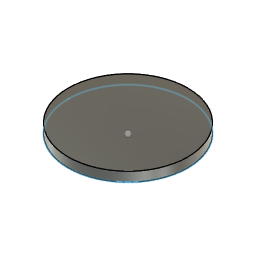
token (Autodesk Fusion 360 design; units mm, degrees)
Autodesk Fusion 360 part; units mm, degrees
sketch "sketch 483" plane through (0, 0, 100) normal (0, 0, 1) x (-1, 0, 0)
  circle A0 centre (0, 0) radius 19
extrude "Extrude1" add sketch "sketch 483" along normal blind 1
sketch "Sketch1" plane through (0, 0, 101) normal (0, 0, 1) x (-1, 0, 0)
  circle A0 centre (0, 0) radius 19
  circle A1 centre (0, 0) radius 13
  dimension "d134" = 26
  constraint concentric A0 A1
  measures "d134" diameter of A1
extrude "Extrude2" add sketch "Sketch1" along normal blind 1
sketch "Sketch2" plane through (0, 0, 102) normal (0, 0, 1) x (-1, 0, 0)
  circle A0 centre (0, 0) radius 13
  circle A1 centre (0, 0) radius 19
  circle A2 centre (0, 0) radius 19
  constraint concentric A0 A2
extrude "Extrude3" add sketch "Sketch2" along normal blind 1 contours A0 | A1 A2
